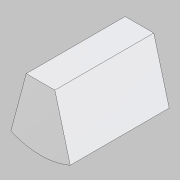
# Autodesk Inventor part: CA001
Saved by Autodesk Inventor 2017 (Build 210142000, 142)
## iProperties
Created: 2017-06-04
Part Number: CA001
Material: ABS Plastic
Document SubType Name: Modeling
Designer: Zach
Density: 1.06 g/cm^3
Appearance: CR White
Author: Zach
Autodesk Inventor part; units mm, degrees
ref_plane "YZ Plane" through (0, 0, 0) normal (1, 0, 0) x (0, 1, 0)
ref_plane "XZ Plane" through (0, 0, 0) normal (0, 1, 0) x (-1, 0, 0)
ref_plane "XY Plane" through (0, 0, 0) normal (0, 0, 1) x (1, 0, 0)
sketch "Sketch1" plane through (0, 0, 0) normal (0, 0, 1) x (1, 0, 0)
  line L0 (0, 0) -> (180, 0)
  line L1 (180, 0) -> (133.4126, 173.8666)
  line L2 (46.5874, 173.8666) -> (0, 0)
  line L3 (46.5874, 173.8666) -> (133.4126, 173.8666)
  dimension "d0" = 180
  dimension "d1" = 180
  dimension "d2" = 75
  dimension "d8" = 75
  constraints: 8 end point, 2 horizontal
  measures "d0" distance of L0.start L0.end
  measures "d1" distance of L1.end L0.end
  measures "d2" angle of L1 L0
  measures "d8" angle of L0 L2
extrude "Extrusion1" add sketch "Sketch1" along normal blind 300
sketch "Sketch2" plane through (0, 0, 300) normal (0, 0, 1) x (1, 0, 0)
  circle A0 centre (90, 206.2159) radius 225 construction
  line L0 (0, 0) -> (180, 0) projected
  arc A1 (0, 0) -> (180, 0) centre (90, 206.2159) ccw
  line L1 (180, 0) -> (127.5964, 195.5729) projected
  line L2 (180, 0) -> (0, 0)
  point P0 (46.5874, 173.8666)
  dimension "d5" = 450
  constraints: 4 point on circle, 2 centre point, 2 end point, 1 concentric, 1 horizontal
  measures "d5" diameter of A0
extrude "Extrusion2" add sketch "Sketch2" against normal blind 300
body "Solid1"
